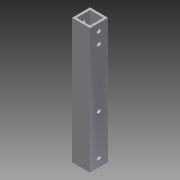
# Autodesk Inventor part: Chassis V1.500 Part3
Saved by Autodesk Inventor 2013 (Build 170138000, 138)
## iProperties
Created: 2013-01-05
Part Number: Chassis V1.500 Part3
Material: Aluminum 6061
Document SubType Name: Modeling
Designer: Moses
Density: 2.71 g/cm^3
Mass: 133.645 g
Surface Area: 321.563 cm^2
Volume: 49.3153 cm^3
Author: Moses
Autodesk Inventor part; units mm, degrees
ref_plane "YZ Plane" through (0, 0, 0) normal (1, 0, 0) x (0, 1, 0)
ref_plane "XZ Plane" through (0, 0, 0) normal (0, 1, 0) x (-1, 0, 0)
ref_plane "XY Plane" through (0, 0, 0) normal (0, 0, 1) x (1, 0, 0)
sketch "Sketch1" plane through (0, 0, 0) normal (0, 1, 0) x (-1, 0, 0)
  line L0 (0, 25.4) -> (25.4, 25.4)
  line L1 (25.4, 25.4) -> (25.4, 0)
  line L2 (25.4, 0) -> (0, 0)
  line L3 (0, 0) -> (0, 25.4)
  line L4 (22.225, 22.225) -> (3.175, 22.225)
  line L5 (3.175, 22.225) -> (3.175, 3.175)
  line L6 (3.175, 3.175) -> (22.225, 3.175)
  line L7 (22.225, 3.175) -> (22.225, 22.225)
  dimension "d0" = 25.4
  dimension "d1" = 25.4
  dimension "d2" = 3.175
  constraints: 16 end point, 4 parallel, 2 perpendicular, 1 coincident, 1 horizontal, 3 other
  measures "d0" distance of L1.end L2.end
  measures "d1" distance of L0.end L1.end
  measures "d2" distance between parallel lines of L0 L4
extrude "Extrusion1" add sketch "Sketch1" along normal blind 177.8
sketch "Sketch2" plane through (-25.4, 0, 0) normal (-1, 0, 0) x (0, 0, 1)
  line L0 (25.4, 0) -> (0, 0) projected
  line L1 (0, 177.8) -> (25.4, 177.8) projected
  line L2 (12.7, 0) -> (12.7, 177.8) construction
  circle A0 centre (12.7, 12.7) radius 3.302
  circle A1 centre (12.7, 69.85) radius 3.302
  circle A2 centre (12.7, 25.4) radius 3.302
  circle A3 centre (12.7, 168.275) radius 3.302 projected
  circle A4 centre (12.7, 152.4) radius 3.302 projected
  dimension "d16" = 6.604
  dimension "d17" = 6.604
  dimension "d18" = 107.95
  dimension "d19" = 6.604
  dimension "d20" = 12.7
  dimension "d21" = 12.7
  constraints: 3 centre point, 3 point on line, 2 end point, 2 midpoint
  measures "d16" diameter of A0
  measures "d17" diameter of A1
  measures "d18" distance from line of L1 A1.centre
  measures "d19" diameter of A2
  measures "d20" distance of A0.centre A2.centre
  measures "d21" distance from line of L0 A0.centre
extrude "Extrusion2" cut sketch "Sketch2" against normal blind 25.4 contours A0 | A1 | A3 | A4
equation "\"d19\" = d16"
equation "\"d21\" = d20"
body "Solid1"
